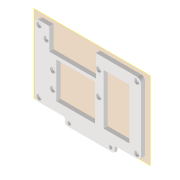
# Autodesk Inventor part: 11_Wellplatespacer
Saved by Autodesk Inventor 2022 (Build 260153000, 153)
## iProperties
Created: 2023-01-07
Part Number: 11_Wellplatespacer
Material: Generisch
Document SubType Name: Modeling
Designer: diederichbenedict
Density: 1 g/cm^3
Appearance: Vorgabe
Author: diederichbenedict
Autodesk Inventor part; units mm, degrees
ref_plane "YZ Plane" through (0, 0, 0) normal (1, 0, 0) x (0, 1, 0)
ref_plane "XZ Plane" through (0, 0, 0) normal (0, 1, 0) x (-1, 0, 0)
ref_plane "XY Plane" through (0, 0, 0) normal (0, 0, 1) x (1, 0, 0)
ref_plane "Arbeitsebene1" through (0, 0, 0) normal (0, 0, 1) x (1, 0, 0)
sketch "Skizze1" plane through (0, 0, 0) normal (0, 0, 1) x (1, 0, 0)
  line L0 (8.6, 2.25) -> (8.6, -41.35) projected
  line L1 (8.6, -41.35) -> (-37.9, -41.35) projected
  line L2 (-37.9, -41.35) -> (-37.9, 2.25) projected
  line L3 (-37.9, 2.25) -> (8.6, 2.25) projected
  line L4 (9.6, 6.25) -> (-46.4, 6.25) projected
  line L5 (-46.4, 32.25) -> (-46.4, 6.25) projected
  line L6 (9.6, 32.25) -> (-46.4, 32.25) projected
  line L7 (9.6, 6.25) -> (9.6, 32.25) projected
  circle A0 centre (13.1, -11.2637) radius 1.4 projected
  circle A1 centre (-42.4, -11.2637) radius 1.4 projected
  circle A2 centre (-42.4, -31.25) radius 1.4 projected
  line L8 (18.9, -41.35) -> (18.9, 19.75) projected
  line L9 (18.9, 19.75) -> (58.9, 19.75) projected
  line L10 (58.9, 19.75) -> (58.9, 19.25) projected
  line L11 (58.9, 19.25) -> (55.9, 19.25) projected
  line L12 (55.9, 17.6031) -> (55.9, 19.25) projected
  line L13 (63.9, 17.6031) -> (55.9, 17.6031) projected
  line L14 (63.9, 27.75) -> (63.9, 17.6031) projected
  arc A3 (63.9, 27.75) -> (58.9, 32.75) centre (58.9, 27.75) ccw projected
  line L15 (58.9, 32.75) -> (-58.9, 32.75) projected
  arc A4 (-58.9, 32.75) -> (-63.9, 27.75) centre (-58.9, 27.75) ccw projected
  line L16 (-63.9, -47.75) -> (-63.9, 27.75) projected
  arc A5 (-63.9, -47.75) -> (-58.9, -52.75) centre (-58.9, -47.75) ccw projected
  line L17 (-58.9, -52.75) -> (58.9, -52.75) projected
  arc A6 (58.9, -52.75) -> (63.9, -47.75) centre (58.9, -47.75) ccw projected
  line L18 (63.9, -47.75) -> (63.9, 0.8969) projected
  line L19 (55.9, 0.8969) -> (63.9, 0.8969) projected
  line L20 (55.9, -0.75) -> (55.9, 0.8969) projected
  line L21 (58.9, -0.75) -> (55.9, -0.75) projected
  line L22 (58.9, -0.75) -> (58.9, -1.25) projected
  line L23 (58.9, -1.25) -> (49.9, -1.25) projected
  line L24 (49.9, -1.25) -> (49.9, -41.35) projected
  line L25 (49.9, -41.35) -> (18.9, -41.35) projected
  circle A7 centre (13.1, 17.25) radius 1.4 projected
  circle A8 centre (-50.2191, 17.25) radius 1.4 projected
  line L26 (63.9, 17.6031) -> (63.9, 0.8969)
  line L27 (49.9, -1.25) -> (49.9, 19.75)
  line L28 (18.9, 6.25) -> (9.6, 6.25)
  line L29 (9.6, 6.25) -> (9.6, 2.25)
  line L30 (9.6, 2.25) -> (8.6, 2.25)
  line L31 (-37.9, 2.25) -> (-46.4, 2.25)
  line L32 (-46.4, 2.25) -> (-46.4, 6.25)
  line L33 (9.6, 32.25) -> (9.6, 32.75)
  line L34 (-46.4, 32.25) -> (-46.4, 32.75)
  circle A9 centre (58.9, 27.75) radius 1.4
  circle A10 centre (58.9, -47.75) radius 1.4
  circle A11 centre (-58.9, -47.75) radius 1.4
  circle A12 centre (-58.9, 27.75) radius 1.4
  point P0 (0, 0)
  dimension "d0" = 2.8
  dimension "d1" = 2.8
  dimension "d2" = 2.8
  dimension "d3" = 2.8
  constraints: 18 end point, 7 point on line, 4 centre point, 4 coincident, 3 perpendicular, 2 vertical, 1 parallel
  measures "d0" diameter of A9
  measures "d1" diameter of A10
  measures "d2" diameter of A11
  measures "d3" diameter of A12
extrude "Extrusion1" add sketch "Skizze1" along normal blind 5 contours L30 L29 L28 L8 L25 L24 L23 L22 L21 L20 L19 L18 A6 L17 A5 L16 A4 L15 L34 L5 L32 L31 L2 L1 L0 | L3 L31 L32 L4 L29 L30 | L7 L33 L15 A3 L14 L13 L12 L11 L10 L9 L8 L28 | L9 L10 L11 L12 L13 L26 L19 L20 L21 L22 L23 L27
sketch "Skizze2" plane through (0, 0, 5) normal (0, 0, 1) x (1, 0, 0)
  line L0 (-58.9, -52.75) -> (58.9, -52.75) projected
  line L1 (32.321, -52.75) -> (-27.679, -52.75)
  line L2 (-27.679, -52.75) -> (-27.679, -60.75)
  line L3 (-27.679, -60.75) -> (32.321, -60.75)
  line L4 (32.321, -60.75) -> (32.321, -52.75)
  circle A0 centre (27.321, -56.75) radius 2.25
  circle A1 centre (-22.679, -56.75) radius 2.25
  point P0 (0, 0)
  dimension "d6" = 60
  dimension "d7" = 8
  dimension "d8" = 4.5
  dimension "d9" = 4.5
  dimension "d10" = 5
  dimension "d11" = 50
  constraints: 8 end point, 2 centre point, 2 parallel, 1 horizontal, 1 perpendicular, 1 point on line
  measures "d6" distance of L3.end L2.end
  measures "d7" distance of L2.end L1.end
  measures "d8" diameter of A0
  measures "d9" diameter of A1
  measures "d10" distance from line of A0.centre L4
  measures "d11" distance of A1.centre A0.centre
extrude "Extrusion2" add sketch "Skizze2" against normal blind 3
fillet "Rundung1" radius 2 4 edges at (32.321, -60.75, 3.5) (32.321, -52.75, 3.5) (-27.679, -52.75, 3.5) (-27.679, -60.75, 3.5)
sketch "Skizze3" plane through (0, 0, 5) normal (0, 0, 1) x (1, 0, 0)
  arc A0 (-27.679, -58.75) -> (-25.679, -60.75) centre (-25.679, -58.75) ccw projected
  line L0 (-25.679, -60.75) -> (30.321, -60.75) projected
  arc A1 (30.321, -60.75) -> (32.321, -58.75) centre (30.321, -58.75) ccw projected
  line L1 (32.321, -58.75) -> (32.321, -54.75) projected
  arc A2 (34.321, -52.75) -> (32.321, -54.75) centre (34.321, -54.75) ccw projected
  line L2 (34.321, -52.75) -> (58.9, -52.75) projected
  arc A3 (58.9, -52.75) -> (63.9, -47.75) centre (58.9, -47.75) ccw projected
  line L3 (63.9, -47.75) -> (63.9, 27.75) projected
  arc A4 (63.9, 27.75) -> (58.9, 32.75) centre (58.9, 27.75) ccw projected
  line L4 (58.9, 32.75) -> (9.6, 32.75) projected
  line L5 (9.6, 32.75) -> (9.6, 6.25) projected
  line L6 (9.6, 6.25) -> (-46.4, 6.25) projected
  line L7 (-46.4, 6.25) -> (-46.4, 32.75) projected
  line L8 (-46.4, 32.75) -> (-58.9, 32.75) projected
  arc A5 (-58.9, 32.75) -> (-63.9, 27.75) centre (-58.9, 27.75) ccw projected
  line L9 (-63.9, 27.75) -> (-63.9, -47.75) projected
  arc A6 (-63.9, -47.75) -> (-58.9, -52.75) centre (-58.9, -47.75) ccw projected
  line L10 (-58.9, -52.75) -> (-29.679, -52.75) projected
  arc A7 (-27.679, -54.75) -> (-29.679, -52.75) centre (-29.679, -54.75) ccw projected
  line L11 (-27.679, -54.75) -> (-27.679, -58.75) projected
  circle A8 centre (13.1, 17.25) radius 1.4 projected
  circle A9 centre (58.9, 27.75) radius 1.4 projected
  circle A10 centre (13.1, -11.2637) radius 1.4 projected
  circle A11 centre (-42.4, -11.2637) radius 1.4 projected
  circle A12 centre (-42.4, -31.25) radius 1.4 projected
  circle A13 centre (-50.2191, 17.25) radius 1.4 projected
  circle A14 centre (-58.9, 27.75) radius 1.4 projected
  circle A15 centre (-58.9, -47.75) radius 1.4 projected
  circle A16 centre (58.9, -47.75) radius 1.4 projected
  line L12 (8.6, 2.25) -> (8.6, -41.35) projected
  line L13 (8.6, -41.35) -> (-37.9, -41.35) projected
  line L14 (-37.9, -41.35) -> (-37.9, 2.25) projected
  line L15 (-37.9, 2.25) -> (8.6, 2.25) projected
  line L16 (18.9, -41.35) -> (18.9, 19.75) projected
  line L17 (18.9, 19.75) -> (49.9, 19.75) projected
  line L18 (49.9, 19.75) -> (49.9, -41.35) projected
  line L19 (49.9, -41.35) -> (18.9, -41.35) projected
  circle A17 centre (-22.679, -56.75) radius 2.25 projected
  circle A18 centre (27.321, -56.75) radius 2.25 projected
  point P0 (0, 0)
hole "Bohrung1" at (58.9, -47.75, 5) at (-58.9, -47.75, 5) at (-42.4, -31.25, 5) at (-42.4, -11.2637, 5) at (-50.2191, 17.25, 5) at (-58.9, 27.75, 5) at (13.1, -11.2637, 5) at (13.1, 17.25, 5) at (58.9, 27.75, 5) direction (0, 0, -1) diameter 2.9 end through all counterbore diameter 6.5 counterbore depth 3
ref_plane "Arbeitsebene2" through (55.9, -6.9963, -17.125) normal (-1, 0, 0) x (0, 0, 1)
sketch "Skizze4" plane through (49.9, -41.35, 0) normal (-1, 0, 0) x (0, 0, 1)
  line L0 (-10, 60) -> (0, 60)
  line L1 (-7.125, 40.6) -> (0, 40.6) projected
  line L2 (-17.125, 59.1) -> (-17.125, 50.6) projected
  line L3 (1.375, 40.6) -> (-15.625, 40.6)
  line L4 (-17.125, 42.1) -> (-17.125, 59.1)
  line L5 (-15.625, 60.6) -> (1.375, 60.6)
  line L6 (2.875, 59.1) -> (2.875, 42.1)
  line L7 (2.875, 40.6) -> (-17.125, 60.6) construction
  line L8 (-17.125, 40.6) -> (2.875, 60.6) construction
  arc A0 (-15.625, 60.6) -> (-17.125, 59.1) centre (-15.625, 59.1) ccw
  arc A1 (2.875, 59.1) -> (1.375, 60.6) centre (1.375, 59.1) ccw
  arc A2 (1.375, 40.6) -> (2.875, 42.1) centre (1.375, 42.1) ccw
  arc A3 (-17.125, 42.1) -> (-15.625, 40.6) centre (-15.625, 42.1) ccw
  arc A4 (-9, 49.9344) -> (-9, 51.2656) centre (-7.125, 50.6) ccw projected
  point P0 (0, 41.35)
  point P1 (-7.125, 50.6)
  point P2 (0, 40.6)
  dimension "d22" = 20
  dimension "d23" = 20
  dimension "d24" = 1.5
  constraints: 14 end point, 8 point on circle, 8 point on line, 8 tangent, 4 centre point, 3 equal radius, 2 horizontal, 2 midpoint, 2 parallel, 1 perpendicular, 2 other
  measures "d22" distance of L7.end L8.end
  measures "d23" distance of L8.start L7.end
  measures "d24" radius of A0
extrude "Extrusion3" cut sketch "Skizze4" against normal up to surface (6 mm away)
